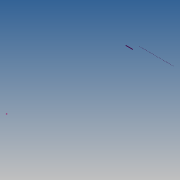
# Autodesk Inventor part: tomites
Saved by Autodesk Inventor 2016 (Build 200138000, 138)
## iProperties
Created: 2017-10-14
Part Number: tomites
Material: Rubber
Document SubType Name: Modeling
Designer: Fauszt
Density: 0.93 g/cm^3
Appearance: Rubber - Black
Mass: 2.28987 g
Surface Area: 36.1126 cm^2
Volume: 2.46222 cm^3
Author: Fauszt
Autodesk Inventor part; units mm, degrees
ref_plane "YZ Plane" through (0, 0, 0) normal (1, 0, 0) x (0, 1, 0)
ref_plane "XZ Plane" through (0, 0, 0) normal (0, 1, 0) x (-1, 0, 0)
ref_plane "XY Plane" through (0, 0, 0) normal (0, 0, 1) x (1, 0, 0)
sketch "Sketch1" plane through (0, 0, 0) normal (0, 0, 1) x (1, 0, 0)
  line L0 (0, 51) -> (3, 51)
  line L1 (3, 53.5) -> (18, 53.5) construction
  line L2 (3, 51) -> (3, 53.5)
  line L3 (0, 53.5) -> (0, 51)
  line L4 (0, 53.5) -> (3, 53.5)
  line L5 (-9, 0) -> (54, 0) construction
  point P0 (0, 0)
  constraints: 12 end point, 3 horizontal, 1 collinear, 1 parallel, 1 vertical, 6 other
revolve "Revolution1" add sketch "Sketch1" angle 360 about axis through (-9, 0, 0) along (1, 0, 0)
body "Solid1"
